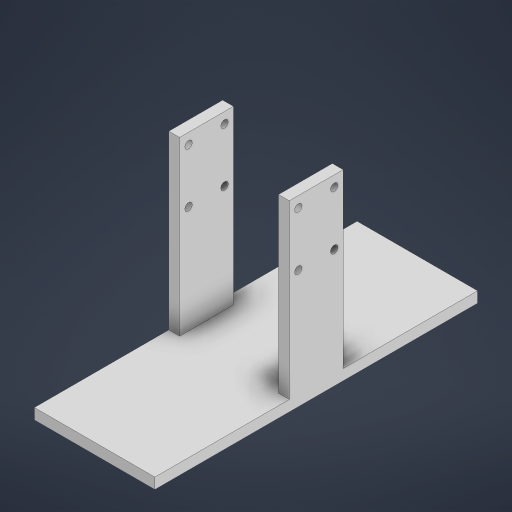
# Autodesk Inventor part: Mounting atas
Saved by Autodesk Inventor 2023.6 (Build 276521000, 521)
## iProperties
Created: 2026-03-05
Part Number: Mounting atas
Material: Generic
Document SubType Name: Modeling
Designer: user
Density: 1 g/cm^3
Appearance: Default
Author: user
Autodesk Inventor part; units mm, degrees
ref_plane "YZ Plane" through (0, 0, 0) normal (1, 0, 0) x (0, 1, 0)
ref_plane "XZ Plane" through (0, 0, 0) normal (0, 1, 0) x (-1, 0, 0)
ref_plane "XY Plane" through (0, 0, 0) normal (0, 0, 1) x (1, 0, 0)
sketch "Sketch1" plane through (0, 0, 0) normal (0, 1, 0) x (-1, 0, 0)
  line L0 (28, 75) -> (-28, 75)
  line L1 (-28, 75) -> (-28, -75)
  line L2 (-28, -75) -> (28, -75)
  line L3 (28, -75) -> (28, 75)
  line L4 (28, 75) -> (-28, -75) construction
  line L5 (-28, 75) -> (28, -75) construction
  point P0 (0, 0)
  dimension "d0" = 56
  dimension "d1" = 150
  constraints: 12 end point, 2 midpoint, 2 parallel, 1 horizontal, 1 perpendicular
  measures "d0" distance between parallel lines of L1 L3
  measures "d1" distance between parallel lines of L2 L0
extrude "Extrusion1" add sketch "Sketch1" along normal blind 5
sketch "Sketch2" plane through (0, 5, 0) normal (0, 1, 0) x (1, 0, 0)
  line L0 (-28, 12.5) -> (-23, 12.5)
  line L1 (-23, 12.5) -> (-23, -12.5)
  line L2 (-23, -12.5) -> (-28, -12.5)
  line L3 (-28, -12.5) -> (-28, 12.5)
  line L4 (-28, 75) -> (-28, -75) projected
  line L5 (0, 0) -> (0, 30.0888)
  line L6 (28, 12.5) -> (23, 12.5)
  line L7 (23, 12.5) -> (23, -12.5)
  line L8 (23, -12.5) -> (28, -12.5)
  line L9 (28, -12.5) -> (28, 12.5)
  point P0 (-28, 0)
  dimension "d4" = 5
  dimension "d5" = 25
  constraints: 18 end point, 4 symmetric about line, 2 midpoint, 2 parallel, 1 horizontal, 1 perpendicular, 1 vertical
  measures "d4" distance between parallel lines of L1 L3
  measures "d5" distance between parallel lines of L0 L2
extrude "Extrusion2" add sketch "Sketch2" along normal blind 80
sketch "Sketch3" plane through (28, 0, 75) normal (1, 0, 0) x (0, 0, -1)
  circle A0 centre (66.65, 55) radius 1.75
  circle A1 centre (66.65, 80) radius 1.75
  circle A2 centre (83.35, 80) radius 1.75
  circle A3 centre (83.35, 55) radius 1.75
  circle A4 centre (66.65, 55) radius 1.75
  circle A5 centre (66.65, 80) radius 1.75
  circle A6 centre (83.35, 80) radius 1.75
  circle A7 centre (83.35, 55) radius 1.75
  line L0 (83.35, 55) -> (66.65, 80)
  line L1 (66.65, 80) -> (66.65, 55)
  line L2 (66.65, 55) -> (83.35, 80)
  line L3 (83.35, 80) -> (83.35, 55)
  line L4 (66.65, 55) -> (83.35, 55)
  line L5 (83.35, 80) -> (66.65, 80)
  line L6 (0, 0) -> (150, 0) projected
  line L7 (150, 0) -> (150, 5) projected
  line L8 (87.5, 5) -> (150, 5) projected
  line L9 (87.5, 5) -> (87.5, 85) projected
  line L10 (62.5, 85) -> (87.5, 85) projected
  line L11 (62.5, 5) -> (62.5, 85) projected
  line L12 (0, 5) -> (62.5, 5) projected
  line L13 (0, 0) -> (0, 5) projected
  line L14 (62.5, 80) -> (87.5, 80)
  line L15 (87.5, 5) -> (87.5, 85) projected
  point P0 (75, 0)
  point P1 (75, 80)
  dimension "d12" = 5
  dimension "d14" = 16.7
  dimension "d15" = 25
  constraints: 14 end point, 8 centre point, 4 coincident, 4 concentric, 2 midpoint, 2 parallel, 2 point on line, 1 perpendicular, 1 vertical
  measures "d12" distance between parallel lines of L10 L14
  measures "d14" distance between parallel lines of L3 L1
  measures "d15" distance of L0.end L1.end
extrude "Extrusion3" cut sketch "Sketch3" against normal through all contours L4 L2 A0 | A0 L1 L4 | L2 L1 A0 | L4 L3 A3 | A3 L0 L4 | L1 L0 A1 | A1 L14 L1 | A3 L3 L0 | L0 L5 A1 | L2 L3 A2 | A2 L5 L2 | A1 L5 L14 | A2 L14 L5 | L3 L14 A2
body "Solid1"
